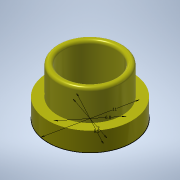
# Autodesk Inventor part: SmaRing_2.5mm_3.0mm_6.8mm
Saved by Autodesk Inventor 2022 (Build 260153000, 153)
## iProperties
Created: 2022-08-18
Part Number: SmaRing_2.5mm_3.0mm_6.8mm
Material: Generic
Document SubType Name: Modeling
Designer: baaij
Density: 1 g/cm^3
Appearance: Yellow
Author: baaij
Autodesk Inventor part; units mm, degrees
ref_plane "YZ Plane" through (0, 0, 0) normal (1, 0, 0) x (0, 1, 0)
ref_plane "XZ Plane" through (0, 0, 0) normal (0, 1, 0) x (-1, 0, 0)
ref_plane "XY Plane" through (0, 0, 0) normal (0, 0, 1) x (1, 0, 0)
sketch "Sketch1" plane through (0, 0, 0) normal (0, 0, 1) x (1, 0, 0)
  circle A0 centre (0, 0) radius 4.25
  circle A1 centre (0, 0) radius 3.5
  circle A2 centre (0, 0) radius 5.5
  circle A3 centre (0, 0) radius 3.4
  dimension "d0" = 8.5
  dimension "d1" = 7
  dimension "d2" = 11
  dimension "d23" = 6.8
  constraints: 4 centre point, 4 coincident
  measures "d0" diameter of A0
  measures "d1" diameter of A1
  measures "d2" diameter of A2
  measures "d23" diameter of A3
extrude "Extrusion1" add sketch "Sketch1" along normal blind 2.5 contours A2
extrude "Extrusion6" add sketch "Sketch1" along normal blind 6.5 contours A0 | A1
fillet "Fillet4" radius 0.4 2 edges at (-3.4, 0, 6.5) (-4.25, 0, 6.5)
extrude "Extrusion13" cut sketch "Sketch1" along normal blind 1.5 contours A1
body "Solid1"
